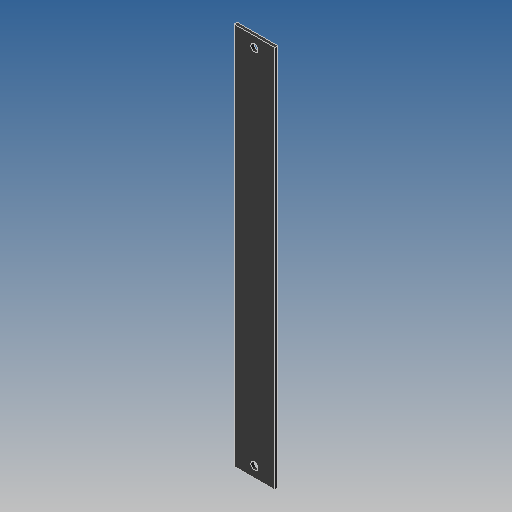
# Autodesk Inventor part: Rotation Resistor-01
Saved by Autodesk Inventor 2018 (Build 220112000, 112)
## iProperties
Created: 2018-02-23
Part Number: Rotation Resistor-01
Material: Generic
Document SubType Name: Modeling
Designer: 232963
Density: 1 g/cm^3
Appearance: Default
Mass: 10.8053 g
Surface Area: 123.742 cm^2
Volume: 10.8053 cm^3
Author: 232963
Autodesk Inventor part; units mm, degrees
ref_plane "YZ Plane" through (0, 0, 0) normal (1, 0, 0) x (0, 1, 0)
ref_plane "XZ Plane" through (0, 0, 0) normal (0, 1, 0) x (-1, 0, 0)
sketch "Sketch1" plane through (0, 0, 0) normal (0, 0, 1) x (1, 0, 0)
  line L0 (-19.7981, 13.2031) -> (4.8082, 13.2031)
  line L1 (4.8082, 13.2031) -> (4.8082, -218.5719)
  line L2 (4.8082, -218.5719) -> (-19.7981, -218.5719)
  line L3 (-19.7981, -218.5719) -> (-19.7981, 13.2031)
  point P0 (0, 0)
  dimension "d0" = 231.775
  dimension "d1" = 24.6062
  constraints: 8 end point, 2 parallel, 1 horizontal, 1 perpendicular
  measures "d0" distance of L0.end L1.end
  measures "d1" distance of L0.start L0.end
extrude "Extrusion1" add sketch "Sketch1" along normal blind 1.905
sketch "Sketch2" plane through (0, 0, 1.905) normal (0, 0, 1) x (1, 0, 0)
  line L0 (4.8082, 13.2031) -> (-19.7981, 13.2031) projected
  line L1 (-7.4949, 13.2031) -> (-7.4949, -18.5655)
  line L2 (-19.7981, 13.2031) -> (-19.7981, -218.5719) projected
  line L3 (4.8082, -218.5719) -> (4.8082, 13.2031) projected
  line L4 (-19.7981, 6.8531) -> (4.8082, 6.8531)
  point P0 (0, 0)
  point P1 (-7.4949, 6.8531)
  point P2 (-7.4949, 6.8531)
  point P3 (-7.4949, 6.8531)
  dimension "d4" = 12.3031
  dimension "d6" = 6.35
  constraints: 4 end point, 2 coincident, 2 midpoint, 2 point on line, 1 perpendicular, 1 vertical
  measures "d4" distance between parallel lines of L2 L1
  measures "d6" distance between parallel lines of L0 L4
hole "Hole1" at (-7.4949, 6.8531, 1.905) direction (0, 0, -1) diameter 4.445 end through all
sketch "Sketch3" plane through (0, 0, 1.905) normal (0, 0, 1) x (1, 0, 0)
  line L0 (4.8082, 13.2031) -> (4.8082, -218.5719) projected
  line L1 (4.8082, -102.6844) -> (-19.7981, -102.6844)
  line L2 (-19.7981, -218.5719) -> (-19.7981, 13.2031) projected
  line L3 (4.8082, 13.2031) -> (-19.7981, 13.2031) projected
  line L4 (4.8082, -218.5719) -> (4.8082, 13.2031) projected
  point P0 (0, 0)
  dimension "d14" = 231.775
  dimension "d15" = 115.8875
  constraints: 2 end point, 2 midpoint, 1 parallel, 1 perpendicular
  measures "d14" distance of L0.start L0.end
  measures "d15" distance between parallel lines of L3 L1
ref_plane "Work Plane1" through (-19.7981, -102.6844, 0) normal (0, 1, 0) x (1, 0, 0)
mirror "Mirror1" about plane through (-19.7981, -102.6844, 0) normal (0, 1, 0) of "Hole1"
equation "\"d15\" = 0.5 * d14"
body "Solid1"
